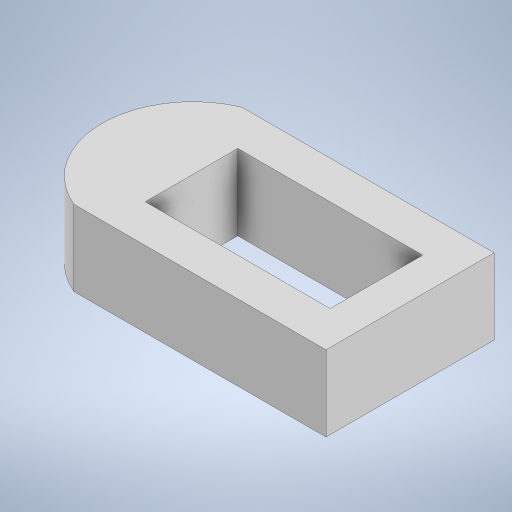
# Autodesk Inventor part: Sensor
Saved by Autodesk Inventor 2024 (Build 280153000, 153)
## iProperties
Created: 2023-07-03
Part Number: Sensor
Material: Generic
Document SubType Name: Modeling
Designer: janro
Density: 1 g/cm^3
Appearance: Default
Author: janro
Autodesk Inventor part; units mm, degrees
ref_plane "YZ Plane" through (0, 0, 0) normal (1, 0, 0) x (0, 1, 0)
ref_plane "XZ Plane" through (0, 0, 0) normal (0, 1, 0) x (-1, 0, 0)
ref_plane "XY Plane" through (0, 0, 0) normal (0, 0, 1) x (1, 0, 0)
sketch "Sketch1" plane through (0, 0, 0) normal (0, 1, 0) x (-1, 0, 0)
  line L0 (-110, 55) -> (110, 55)
  line L1 (110, 55) -> (110, -55)
  line L2 (110, -55) -> (-110, -55)
  line L3 (-110, -55) -> (-110, 55)
  line L4 (-110, 55) -> (110, -55) construction
  line L5 (110, 55) -> (-110, -55) construction
  line L6 (-150, 100) -> (150, 100)
  line L7 (150, 100) -> (150, -100)
  line L8 (150, -100) -> (-150, -100)
  line L9 (-150, -100) -> (-150, 100)
  line L10 (-150, 100) -> (150, -100) construction
  line L11 (150, 100) -> (-150, -100) construction
  arc A0 (150, -100) -> (150, 100) centre (108.3333, 0) ccw
  point P0 (0, 0)
  dimension "d0" = 220
  dimension "d1" = 110
  dimension "d2" = 300
  dimension "d3" = 200
  constraints: 24 end point, 4 midpoint, 4 parallel, 2 horizontal, 2 perpendicular, 2 point on circle, 1 centre point
  measures "d0" distance of L1.end L2.end
  measures "d1" distance of L0.end L1.end
  measures "d2" distance of L7.end L8.end
  measures "d3" distance of L6.end L7.end
extrude "Extrusion1" add sketch "Sketch1" along normal blind 90
body "Solid1"
